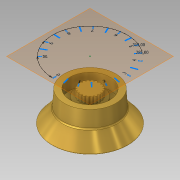
# Autodesk Inventor part: Knob
Saved by Autodesk Inventor 2016 (Build 200138000, 138)
## iProperties
Created: 2018-09-08
Part Number: Knob
Material: Generic
Document SubType Name: Modeling
Designer: Pedro Mendonça
Density: 1 g/cm^3
Appearance: Gold - Metal(1)
Author: Pedro Mendonça
Autodesk Inventor part; units mm, degrees
ref_plane "YZ Plane" through (0, 0, 0) normal (1, 0, 0) x (0, 1, 0)
ref_plane "XZ Plane" through (0, 0, 0) normal (0, 1, 0) x (-1, 0, 0)
sketch "Sketch1" plane through (0, 0, 0) normal (1, 0, 0) x (0, 1, 0)
  line L0 (0, 0) -> (0, 12.45)
  line L1 (0, 12.45) -> (8.7, 12.45)
  line L2 (8.7, 12.45) -> (9.2, 4.8665)
  line L3 (0, 0) -> (13.15, 0)
  line L4 (13.15, 0) -> (9.2, 4.8665)
  line L5 (0, -2.49) -> (0, 14.94) projected
  dimension "d5" = 12.45
  dimension "d6" = 8.7
  dimension "d7" = 7.6
  dimension "d8" = 13.15
  dimension "d10" = 9.2
  constraints: 10 end point, 1 horizontal, 1 perpendicular, 1 vertical
  measures "d5" distance of L0.start L0.end
  measures "d6" distance of L0.end L1.end
  measures "d7" distance of L1.end L2.end
  measures "d8" distance of L0.start L3.end
  measures "d10" distance from line of L2.end L0
revolve "Revolution1" add sketch "Sketch1" angle 360 about axis through (0, 0, -10) along (0, 0, 1)
sketch "Sketch2" plane through (0, 0, 0) normal (1, 0, 0) x (0, 1, 0)
  line L0 (-11.15, 0) -> (-7.2104, 4.8749)
  line L1 (-7.2173, 4.8665) -> (-6.8225, 10.8535)
  line L2 (-6.8225, 10.8535) -> (-4.8225, 10.8535)
  line L3 (-4.8225, 10.8535) -> (-4.8225, 0)
  line L4 (-11.15, 0) -> (-4.8225, 0)
  line L5 (-13.15, 0) -> (13.15, 0) projected
  line L6 (-11.15, 0) -> (-7.2173, 4.8665)
  line L7 (-6.8225, 10.8535) -> (-4.8225, 10.8535)
  line L8 (-4.8225, 0) -> (-11.15, 0)
  line L9 (0, -2.49) -> (0, 14.94) projected
  point P0 (0, 0)
  dimension "d14" = 6
  dimension "d15" = 2
  constraints: 16 end point, 2 horizontal, 2 parallel, 1 collinear
  measures "d14" distance of L1.start L1.end
  measures "d15" distance of L1.end L2.end
revolve "Revolution2" cut sketch "Sketch2" angle 360 about axis through (0, 0, -10) along (0, 0, 1)
sketch "Sketch3" plane through (0, 0, 0) normal (0, 0, -1) x (-1, 0, 0)
  circle A0 centre (0, 0) radius 3.125
  dimension "d17" = 6.25
  constraints: 1 centre point, 1 coincident
  measures "d17" diameter of A0
extrude "Extrusion1" cut sketch "Sketch3" against normal blind 8
sketch "Sketch4" plane through (0, 0, 0) normal (0, 0, -1) x (-1, 0, 0)
  circle A0 centre (0, 0) radius 3.125 projected
  circle A1 centre (0, -3.125) radius 0.485
  circle A2 centre (0.9657, -2.9721) radius 0.485
  circle A3 centre (1.8368, -2.5282) radius 0.485
  circle A4 centre (2.5282, -1.8368) radius 0.485
  circle A5 centre (2.9721, -0.9657) radius 0.485
  circle A6 centre (3.125, 0) radius 0.485
  circle A7 centre (2.9721, 0.9657) radius 0.485
  circle A8 centre (2.5282, 1.8368) radius 0.485
  circle A9 centre (1.8368, 2.5282) radius 0.485
  circle A10 centre (0.9657, 2.9721) radius 0.485
  circle A11 centre (0, 3.125) radius 0.485
  circle A12 centre (-0.9657, 2.9721) radius 0.485
  circle A13 centre (-1.8368, 2.5282) radius 0.485
  circle A14 centre (-2.5282, 1.8368) radius 0.485
  circle A15 centre (-2.9721, 0.9657) radius 0.485
  circle A16 centre (-3.125, 0) radius 0.485
  circle A17 centre (-2.9721, -0.9657) radius 0.485
  circle A18 centre (-2.5282, -1.8368) radius 0.485
  circle A19 centre (-1.8368, -2.5282) radius 0.485
  circle A20 centre (-0.9657, -2.9721) radius 0.485
  dimension "d20" = 0.97
  dimension "d23" = 360
  constraints: 20 centre point, 1 vertical alignment, 42 other
  measures "d20" diameter of A1
extrude "Extrusion2" cut sketch "Sketch4" against normal blind 8 contours A0 A6 | A0 A6 | A7 A0 | A0 A7 | A5 A0 | A0 A5 | A8 A0 | A0 A8 | A4 A0 | A0 A4 | A9 A0 | A0 A9 | A3 A0 | A0 A3 | A10 A0 | A0 A10 | A2 A0 | A0 A2 | A11 A0 | A0 A11 | A1 A0 | A0 A1 | A12 A0 | A0 A12 | A20 A0 | A0 A20 | A13 A0 | A0 A13 | A19 A0 | A0 A19 | A14 A0 | A0 A14 | A18 A0 | A0 A18 | A15 A0 | A0 A15 | A17 A0 | A0 A17 | A16 A0 | A0 A16
fillet "Fillet1" radius 1 1 edges at (0, -9.2, 4.8665)
fillet "Fillet3" radius 0.1 1 edges at (0, -13.15, 0)
sketch "Sketch7" plane through (0, 0, 12.45) normal (0, 0, 1) x (1, 0, 0)
  circle A0 centre (0, 0) radius 10
  dimension "d95" = 20
  constraints: 1 centre point, 1 coincident
  measures "d95" diameter of A0
extrude "Extrusion4" cut sketch "Sketch7" against normal blind 2
sketch "Sketch8" plane through (0, 0, 0) normal (0, 0, -1) x (-1, 0, 0)
  circle A0 centre (0, 0) radius 4.8225
  constraints: 1 centre point, 1 coincident
extrude "Extrusion5" cut sketch "Sketch8" against normal blind 2.5
sketch "Sketch9" plane through (0, 0, 10.45) normal (0, 0, 1) x (1, 0, 0)
  circle A0 centre (0, 0) radius 4.8225 projected
  arc A1 (-1.4235, 2.7819) -> (-2.2059, 2.2135) centre (-1.8368, 2.5282) ccw projected
  arc A2 (-0.4942, 3.0857) -> (-1.4139, 2.7868) centre (-0.9657, 2.9721) ccw projected
  arc A3 (0.4835, 3.0874) -> (-0.4835, 3.0874) centre (0, 3.125) ccw projected
  arc A4 (1.4139, 2.7868) -> (0.4942, 3.0857) centre (0.9657, 2.9721) ccw projected
  arc A5 (2.2059, 2.2135) -> (1.4235, 2.7819) centre (1.8368, 2.5282) ccw projected
  arc A6 (2.7819, 1.4235) -> (2.2135, 2.2059) centre (2.5282, 1.8368) ccw projected
  arc A7 (3.0857, 0.4942) -> (2.7868, 1.4139) centre (2.9721, 0.9657) ccw projected
  arc A8 (3.0874, -0.4835) -> (3.0874, 0.4835) centre (3.125, 0) ccw projected
  arc A9 (2.7868, -1.4139) -> (3.0857, -0.4942) centre (2.9721, -0.9657) ccw projected
  arc A10 (2.2135, -2.2059) -> (2.7819, -1.4235) centre (2.5282, -1.8368) ccw projected
  arc A11 (1.4235, -2.7819) -> (2.2059, -2.2135) centre (1.8368, -2.5282) ccw projected
  arc A12 (0.4942, -3.0857) -> (1.4139, -2.7868) centre (0.9657, -2.9721) ccw projected
  arc A13 (-0.4835, -3.0874) -> (0.4835, -3.0874) centre (0, -3.125) ccw projected
  arc A14 (-1.4139, -2.7868) -> (-0.4942, -3.0857) centre (-0.9657, -2.9721) ccw projected
  arc A15 (-2.2059, -2.2135) -> (-1.4235, -2.7819) centre (-1.8368, -2.5282) ccw projected
  arc A16 (-2.7819, -1.4235) -> (-2.2135, -2.2059) centre (-2.5282, -1.8368) ccw projected
  arc A17 (-3.0857, -0.4942) -> (-2.7868, -1.4139) centre (-2.9721, -0.9657) ccw projected
  arc A18 (-3.0874, 0.4835) -> (-3.0874, -0.4835) centre (-3.125, 0) ccw projected
  arc A19 (-2.7868, 1.4139) -> (-3.0857, 0.4942) centre (-2.9721, 0.9657) ccw projected
  arc A20 (-2.2135, 2.2059) -> (-2.7819, 1.4235) centre (-2.5282, 1.8368) ccw projected
  arc A21 (3.0857, -0.4942) -> (3.0874, -0.4835) centre (0, 0) ccw
  arc A22 (3.0874, 0.4835) -> (3.0857, 0.4942) centre (0, 0) ccw
  arc A23 (2.7868, 1.4139) -> (2.7819, 1.4235) centre (0, 0) ccw
  arc A24 (2.2135, 2.2059) -> (2.2059, 2.2135) centre (0, 0) ccw
  arc A25 (1.4235, 2.7819) -> (1.4139, 2.7868) centre (0, 0) ccw
  arc A26 (0.4942, 3.0857) -> (0.4835, 3.0874) centre (0, 0) ccw
  arc A27 (-0.4835, 3.0874) -> (-0.4942, 3.0857) centre (0, 0) ccw
  arc A28 (-1.4139, 2.7868) -> (-1.4235, 2.7819) centre (0, 0) ccw
  arc A29 (-2.2059, 2.2135) -> (-2.2135, 2.2059) centre (0, 0) ccw
  arc A30 (-2.7819, 1.4235) -> (-2.7868, 1.4139) centre (0, 0) ccw
  arc A31 (-3.0857, 0.4942) -> (-3.0874, 0.4835) centre (0, 0) ccw
  arc A32 (-3.0874, -0.4835) -> (-3.0857, -0.4942) centre (0, 0) ccw
  arc A33 (-2.7868, -1.4139) -> (-2.7819, -1.4235) centre (0, 0) ccw
  arc A34 (-2.2135, -2.2059) -> (-2.2059, -2.2135) centre (0, 0) ccw
  arc A35 (-1.4235, -2.7819) -> (-1.4139, -2.7868) centre (0, 0) ccw
  arc A36 (-0.4942, -3.0857) -> (-0.4835, -3.0874) centre (0, 0) ccw
  arc A37 (0.4835, -3.0874) -> (0.4942, -3.0857) centre (0, 0) ccw
  arc A38 (1.4139, -2.7868) -> (1.4235, -2.7819) centre (0, 0) ccw
  arc A39 (2.2059, -2.2135) -> (2.2135, -2.2059) centre (0, 0) ccw
  arc A40 (2.7819, -1.4235) -> (2.7868, -1.4139) centre (0, 0) ccw
  constraints: 80 point on circle, 20 centre point, 1 coincident
extrude "Extrusion6" cut sketch "Sketch9" against normal blind 2.3
ref_plane "Work Plane2" through (0, 0, 6.15) normal (0, 0, 1) x (1, 0, 0)
sketch "Sketch11" plane through (0, 0, 6.15) normal (0, 0, 1) x (1, 0, 0)
  circle A0 centre (0, 0) radius 7.75
  circle A1 centre (0, 0) radius 4.8212
  dimension "d106" = 15.5
  constraints: 2 centre point, 2 coincident
  measures "d106" diameter of A0
extrude "Extrusion9" add sketch "Sketch11" against normal blind 1
ref_plane "Work Plane3" through (0, 0, 20) normal (0, 0, 1) x (1, 0, 0)
sketch "Sketch12" plane through (0, 0, 20) normal (0, 0, 1) x (1, 0, 0)
  line L0 (12.8, -0.1) -> (11.8, -0.1)
  line L1 (11.8, -0.1) -> (11.8, 0.1)
  line L2 (11.8, 0.1) -> (12.8, 0.1)
  line L3 (12.8, 0.1) -> (12.8, -0.1)
  line L4 (12.8, -0.1) -> (11.8, 0.1) construction
  line L5 (11.8, -0.1) -> (12.8, 0.1) construction
  line L6 (10.4579, 2.6987) -> (12.3897, 3.2163)
  line L7 (12.3897, 3.2163) -> (12.338, 3.4095)
  line L8 (12.338, 3.4095) -> (10.4061, 2.8918)
  line L9 (10.4061, 2.8918) -> (10.4579, 2.6987)
  line L10 (10.9468, 6.6346) -> (10.0957, 6.1096)
  line L11 (10.0957, 6.1096) -> (9.9907, 6.2798)
  line L12 (9.9907, 6.2798) -> (10.8418, 6.8048)
  line L13 (10.8418, 6.8048) -> (10.9468, 6.6346)
  line L14 (10.9468, 6.6346) -> (9.9907, 6.2798) construction
  line L15 (10.0957, 6.1096) -> (10.8418, 6.8048) construction
  line L16 (7.4841, 7.787) -> (8.8566, 9.2418)
  line L17 (8.8566, 9.2418) -> (8.7112, 9.379)
  line L18 (8.7112, 9.379) -> (7.3387, 7.9243)
  line L19 (7.3387, 7.9243) -> (7.4841, 7.787)
  line L20 (5.834, 11.3936) -> (5.3852, 10.5)
  line L21 (5.3852, 10.5) -> (5.2065, 10.5897)
  line L22 (5.2065, 10.5897) -> (5.6553, 11.4834)
  line L23 (5.6553, 11.4834) -> (5.834, 11.3936)
  line L24 (5.834, 11.3936) -> (5.2065, 10.5897) construction
  line L25 (5.3852, 10.5) -> (5.6553, 11.4834) construction
  line L26 (2.2819, 10.5567) -> (2.6863, 12.5153)
  line L27 (2.6863, 12.5153) -> (2.4905, 12.5558)
  line L28 (2.4905, 12.5558) -> (2.086, 10.5971)
  line L29 (2.086, 10.5971) -> (2.2819, 10.5567)
  line L30 (-1.016, 12.76) -> (-0.9288, 11.7638)
  line L31 (-0.9288, 11.7638) -> (-1.1281, 11.7464)
  line L32 (-1.1281, 11.7464) -> (-1.2152, 12.7426)
  line L33 (-1.2152, 12.7426) -> (-1.016, 12.76)
  line L34 (-1.016, 12.76) -> (-1.1281, 11.7464) construction
  line L35 (-0.9288, 11.7638) -> (-1.2152, 12.7426) construction
  line L36 (-3.5998, 10.1829) -> (-4.2839, 12.0623)
  line L37 (-4.2839, 12.0623) -> (-4.4718, 11.9939)
  line L38 (-4.4718, 11.9939) -> (-3.7878, 10.1145)
  line L39 (-3.7878, 10.1145) -> (-3.5998, 10.1829)
  line L40 (-7.5634, 10.3269) -> (-6.9663, 9.5248)
  line L41 (-6.9663, 9.5248) -> (-7.1267, 9.4053)
  line L42 (-7.1267, 9.4053) -> (-7.7238, 10.2075)
  line L43 (-7.7238, 10.2075) -> (-7.5634, 10.3269)
  line L44 (-7.5634, 10.3269) -> (-7.1267, 9.4053) construction
  line L45 (-6.9663, 9.5248) -> (-7.7238, 10.2075) construction
  line L46 (-8.4097, 6.777) -> (-9.9785, 8.0175)
  line L47 (-9.9785, 8.0175) -> (-10.1025, 7.8606)
  line L48 (-10.1025, 7.8606) -> (-8.5337, 6.6201)
  line L49 (-8.5337, 6.6201) -> (-8.4097, 6.777)
  line L50 (-11.8587, 4.8188) -> (-10.9294, 4.4496)
  line L51 (-10.9294, 4.4496) -> (-11.0032, 4.2637)
  line L52 (-11.0032, 4.2637) -> (-11.9326, 4.6329)
  line L53 (-11.9326, 4.6329) -> (-11.8587, 4.8188)
  line L54 (-11.8587, 4.8188) -> (-11.0032, 4.2637) construction
  line L55 (-10.9294, 4.4496) -> (-11.9326, 4.6329) construction
  line L56 (-10.7154, 1.3531) -> (-12.7018, 1.5853)
  line L57 (-12.7018, 1.5853) -> (-12.7251, 1.3867)
  line L58 (-12.7251, 1.3867) -> (-10.7386, 1.1545)
  line L59 (-10.7386, 1.1545) -> (-10.7154, 1.3531)
  line L60 (-12.6229, -2.1242) -> (-11.6381, -1.9506)
  line L61 (-11.6381, -1.9506) -> (-11.6034, -2.1475)
  line L62 (-11.6034, -2.1475) -> (-12.5882, -2.3212)
  line L63 (-12.5882, -2.3212) -> (-12.6229, -2.1242)
  line L64 (-12.6229, -2.1242) -> (-11.6034, -2.1475) construction
  line L65 (-11.6381, -1.9506) -> (-12.5882, -2.3212) construction
  line L66 (-9.8304, -4.4736) -> (-11.643, -5.3189)
  line L67 (-11.643, -5.3189) -> (-11.5585, -5.5001)
  line L68 (-11.5585, -5.5001) -> (-9.7459, -4.6549)
  line L69 (-9.7459, -4.6549) -> (-9.8304, -4.4736)
  line L70 (-9.6284, -8.4347) -> (-8.8814, -7.7699)
  line L71 (-8.8814, -7.7699) -> (-8.7484, -7.9193)
  line L72 (-8.7484, -7.9193) -> (-9.4954, -8.5841)
  line L73 (-9.4954, -8.5841) -> (-9.6284, -8.4347)
  line L74 (-9.6284, -8.4347) -> (-8.7484, -7.9193) construction
  line L75 (-8.8814, -7.7699) -> (-9.4954, -8.5841) construction
  line L76 (-6.0182, -8.9683) -> (-7.1173, -10.6393)
  line L77 (-7.1173, -10.6393) -> (-6.9502, -10.7492)
  line L78 (-6.9502, -10.7492) -> (-5.8511, -9.0782)
  line L79 (-5.8511, -9.0782) -> (-6.0182, -8.9683)
  line L80 (-3.7669, -12.2336) -> (-3.4801, -11.2756)
  line L81 (-3.4801, -11.2756) -> (-3.2885, -11.333)
  line L82 (-3.2885, -11.333) -> (-3.5753, -12.2909)
  line L83 (-3.5753, -12.2909) -> (-3.7669, -12.2336)
  line L84 (-3.7669, -12.2336) -> (-3.2885, -11.333) construction
  line L85 (-3.4801, -11.2756) -> (-3.5753, -12.2909) construction
  line L86 (-0.4141, -10.7925) -> (-0.4722, -12.7917)
  line L87 (-0.4722, -12.7917) -> (-0.2723, -12.7975)
  line L88 (-0.2723, -12.7975) -> (-0.2142, -10.7983)
  line L89 (-0.2142, -10.7983) -> (-0.4141, -10.7925)
  line L90 (3.2163, -12.3897) -> (2.9575, -11.4238)
  line L91 (2.9575, -11.4238) -> (3.1507, -11.372)
  line L92 (3.1507, -11.372) -> (3.4095, -12.338)
  line L93 (3.4095, -12.338) -> (3.2163, -12.3897)
  line L94 (3.2163, -12.3897) -> (3.1507, -11.372) construction
  line L95 (2.9575, -11.4238) -> (3.4095, -12.338) construction
  line L96 (5.3134, -9.4031) -> (6.3134, -11.1351)
  line L97 (6.3134, -11.1351) -> (6.4866, -11.0351)
  line L98 (6.4866, -11.0351) -> (5.4866, -9.3031)
  line L99 (5.4866, -9.3031) -> (5.3134, -9.4031)
  line L100 (8.2731, -8.4146) -> (8.4146, -8.2731)
  line L101 (8.4146, -8.2731) -> (9.1217, -8.9803)
  line L102 (8.9803, -9.1217) -> (8.2731, -8.4146)
  line L103 (8.9803, -9.1217) -> (8.4146, -8.2731) construction
  line L104 (8.2731, -8.4146) -> (9.1217, -8.9803) construction
  line L105 (9.1217, -8.9803) -> (8.9803, -9.1217)
  line L106 (10.4323, -0.3696) -> (10.4323, 0.5179) construction
  line L107 (10.4323, 0.5179) -> (11.6764, 0.5179) construction
  line L108 (11.6764, 0.5179) -> (11.6764, -0.3696) construction
  line L109 (11.6764, -0.3696) -> (10.4323, -0.3696) construction
  line L110 (9.0791, 5.1516) -> (8.6141, 5.9075) construction
  line L111 (8.6141, 5.9075) -> (9.6738, 6.5594) construction
  line L112 (9.6738, 6.5594) -> (10.1388, 5.8035) construction
  line L113 (10.1388, 5.8035) -> (9.0791, 5.1516) construction
  line L114 (4.9856, 9.1713) -> (4.1914, 9.5673) construction
  line L115 (4.1914, 9.5673) -> (4.7465, 10.6807) construction
  line L116 (4.7465, 10.6807) -> (5.5407, 10.2847) construction
  line L117 (5.5407, 10.2847) -> (4.9856, 9.1713) construction
  line L118 (-0.6698, 11.663) -> (-0.5592, 10.4238) construction
  line L119 (-0.5592, 10.4238) -> (-1.4432, 10.3449) construction
  line L120 (-1.4432, 10.3449) -> (-1.5538, 11.5842) construction
  line L121 (-1.5538, 11.5842) -> (-0.6698, 11.663) construction
  line L122 (-5.9233, 8.5956) -> (-6.6358, 8.0664) construction
  line L123 (-6.6358, 8.0664) -> (-7.3775, 9.0653) construction
  line L124 (-7.3775, 9.0653) -> (-6.6651, 9.5944) construction
  line L125 (-6.6651, 9.5944) -> (-5.9233, 8.5956) construction
  line L126 (-10.7041, 4.6794) -> (-9.549, 4.2174) construction
  line L127 (-9.549, 4.2174) -> (-9.8786, 3.3934) construction
  line L128 (-9.8786, 3.3934) -> (-11.0337, 3.8554) construction
  line L129 (-11.0337, 3.8554) -> (-10.7041, 4.6794) construction
  line L130 (-11.5603, -1.6838) -> (-10.3354, -1.4656) construction
  line L131 (-10.3354, -1.4656) -> (-10.1798, -2.3393) construction
  line L132 (-10.1798, -2.3393) -> (-11.4047, -2.5575) construction
  line L133 (-11.4047, -2.5575) -> (-11.5603, -1.6838) construction
  line L134 (-8.9639, -7.4916) -> (-8.035, -6.6639) construction
  line L135 (-8.035, -6.6639) -> (-7.4446, -7.3265) construction
  line L136 (-7.4446, -7.3265) -> (-8.3735, -8.1542) construction
  line L137 (-8.3735, -8.1542) -> (-8.9639, -7.4916) construction
  line L138 (-3.7669, -11.1351) -> (-3.363, -9.8771) construction
  line L139 (-3.363, -9.8771) -> (-2.5697, -10.1318) construction
  line L140 (-2.5697, -10.1318) -> (-2.9736, -11.3898) construction
  line L141 (-2.9736, -11.3898) -> (-3.7669, -11.1351) construction
  line L142 (2.5884, -11.3898) -> (2.2851, -10.1824) construction
  line L143 (2.2851, -10.1824) -> (3.4005, -9.9022) construction
  line L144 (3.4005, -9.9022) -> (3.7038, -11.1097) construction
  line L145 (3.7038, -11.1097) -> (2.5884, -11.3898) construction
  line L146 (7.6666, -8.7681) -> (6.8232, -7.9451) construction
  line L147 (6.8232, -7.9451) -> (8.3823, -6.3474) construction
  line L148 (8.3823, -6.3474) -> (9.2258, -7.1704) construction
  line L149 (9.2258, -7.1704) -> (7.6666, -8.7681) construction
  point P0 (0, 0)
  dimension "d129" = 285
  dimension "d133" = 315
  constraints: 212 end point, 2 parallel, 1 horizontal, 1 perpendicular, 196 other
body "Solid1"
